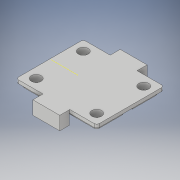
# Autodesk Inventor part: Enclosure_Top V1D5
Saved by Autodesk Inventor 2017 (Build 210142000, 142)
## iProperties
Created: 2017-12-18
Part Number: Enclosure_Top V1D5
Material: Generic
Document SubType Name: Modeling
Designer: Tripl_000
Density: 1 g/cm^3
Appearance: Default
Author: Tripl_000
Autodesk Inventor part; units mm, degrees
ref_plane "YZ Plane" through (0, 0, 0) normal (1, 0, 0) x (0, 1, 0)
ref_plane "XZ Plane" through (0, 0, 0) normal (0, 1, 0) x (-1, 0, 0)
ref_plane "XY Plane" through (0, 0, 0) normal (0, 0, 1) x (1, 0, 0)
sketch "Sketch1" plane through (0, 0, 0) normal (0, 1, 0) x (-1, 0, 0)
  line L0 (28, 23) -> (-28, 23)
  line L1 (-28, 23) -> (-28, -23)
  line L2 (-28, -23) -> (28, -23)
  line L3 (28, -23) -> (28, 23)
  line L4 (28, 23) -> (-28, -23) construction
  line L5 (-28, 23) -> (28, -23) construction
  point P0 (0, 0)
  dimension "d0" = 56
  dimension "d1" = 46
  constraints: 12 end point, 2 midpoint, 2 parallel, 1 horizontal, 1 perpendicular
  measures "d0" distance of L0.start L0.end
  measures "d1" distance of L2.end L0.start
extrude "Extrusion1" add sketch "Sketch1" along normal blind 2.5
sketch "Sketch2" plane through (0, 2.5, 0) normal (0, 1, 0) x (1, 0, 0)
  line L0 (-30, -25) -> (30, -25)
  line L1 (30, -25) -> (30, 25)
  line L2 (30, 25) -> (-30, 25)
  line L3 (-30, 25) -> (-30, -25)
  line L4 (-30, -25) -> (30, 25) construction
  line L5 (30, -25) -> (-30, 25) construction
  point P0 (0, 0)
  dimension "d4" = 50
  dimension "d5" = 60
  constraints: 12 end point, 2 midpoint, 2 parallel, 1 horizontal, 1 perpendicular
  measures "d4" distance of L2.end L0.start
  measures "d5" distance of L0.start L0.end
extrude "Extrusion2" add sketch "Sketch2" along normal blind 2.5
sketch "Sketch3" plane through (28, 0, 23) normal (1, 0, 0) x (0, 0, -1)
  line L0 (19.5, -2.5) -> (26.5, -2.5)
  line L1 (26.5, -2.5) -> (26.5, 2.5)
  line L2 (26.5, 2.5) -> (19.5, 2.5)
  line L3 (19.5, 2.5) -> (19.5, -2.5)
  line L4 (19.5, -2.5) -> (26.5, 2.5) construction
  line L5 (26.5, -2.5) -> (19.5, 2.5) construction
  point P0 (23, 0)
  dimension "d8" = 7
  dimension "d9" = 5
  constraints: 12 end point, 2 midpoint, 2 parallel, 1 horizontal, 1 perpendicular
  measures "d8" distance of L1.end L2.end
  measures "d9" distance of L0.end L1.end
extrude "Extrusion3" cut sketch "Sketch3" against normal through all
sketch "Sketch4" plane through (0, 5, 0) normal (0, 1, 0) x (1, 0, 0)
  line L0 (0, 31.16) -> (0, -35.6529)
  line L1 (-50.8705, 0) -> (45.6531, 0)
  circle A0 centre (-22.5, 17.5) radius 3.683
  circle A1 centre (22.5, 17.5) radius 3.683
  circle A2 centre (-22.5, -17.5) radius 3.683
  circle A3 centre (22.5, -17.5) radius 3.683
  point P0 (0, 0)
  dimension "d12" = 22.5
  dimension "d13" = 17.5
  dimension "d14" = 7.366
  constraints: 4 centre point, 4 end point, 3 symmetric about line, 1 horizontal, 1 vertical, 3 other
  measures "d12" horizontal distance of point (0, 0) A0.centre
  measures "d13" vertical distance of point (0, 0) A0.centre
  measures "d14" diameter of A0
fillet "Fillet1" radius 2 8 edges at (-28, 1.25, 23) (28, 1.25, 23) (28, 1.25, -23) (-28, 1.25, -23) (-30, 3.75, -25) (-30, 3.75, 25) (30, 3.75, 25) (30, 3.75, -25)
extrude "Extrusion5" cut sketch "Sketch4" against normal through all
sketch "Sketch5" plane through (-26, 0, 23) normal (0, 0, 1) x (1, 0, 0)
  line L0 (0, 2.5) -> (52, 2.5) projected
  line L1 (18.5, -2.5) -> (33.5, -2.5)
  line L2 (33.5, -2.5) -> (33.5, 2.5)
  line L3 (33.5, 2.5) -> (18.5, 2.5)
  line L4 (18.5, 2.5) -> (18.5, -2.5)
  line L5 (18.5, -2.5) -> (33.5, 2.5) construction
  line L6 (33.5, -2.5) -> (18.5, 2.5) construction
  point P0 (26, 0)
  dimension "d20" = 15
  constraints: 12 end point, 2 midpoint, 2 parallel, 1 horizontal, 1 perpendicular, 1 point on line
  measures "d20" distance of L1.start L1.end
extrude "Extrusion6" cut sketch "Sketch5" against normal through all
sketch "Sketch6" plane through (-28, 2.5, 25) normal (0, 0, 1) x (1, 0, 0)
  line L0 (20.5, 0) -> (20.5, -2.5) projected
  line L1 (56, 2.5) -> (0, 2.5) projected
  line L2 (20.5, 0) -> (35.5, 0)
  line L3 (35.5, 0) -> (35.5, 2.5)
  line L4 (35.5, 2.5) -> (20.5, 2.5)
  line L5 (20.5, 2.5) -> (20.5, 0)
  point P0 (28, -2.5)
  dimension "d23" = 15
  constraints: 8 end point, 2 parallel, 1 horizontal, 1 perpendicular, 1 point on line
  measures "d23" distance between parallel lines of L3 L5
extrude "Extrusion7" add sketch "Sketch6" along normal blind 10
sketch "Sketch7" plane through (0, 2.5, 0) normal (0, -1, 0) x (1, 0, 0)
  line L0 (-7.5, 25) -> (-7.5, 35) projected
  line L1 (7.5, 25) -> (7.5, 35) projected
  line L2 (-7.5, 35) -> (7.5, 35)
  line L3 (7.5, 35) -> (7.5, 30)
  line L4 (7.5, 30) -> (-7.5, 30)
  line L5 (-7.5, 30) -> (-7.5, 35)
  point P0 (0, 0)
  dimension "d26" = 5
  constraints: 8 end point, 2 parallel, 1 horizontal, 1 midpoint, 1 perpendicular
  measures "d26" distance between parallel lines of L4 L2
extrude "Extrusion8" add sketch "Sketch7" along normal blind 7.5
sketch "Sketch8" plane through (-7.5, 2.5, 25) normal (-1, 0, 0) x (0, 0, 1)
  line L0 (10, 2.5) -> (10, -7.5) projected
  line L1 (0, 2.5) -> (10, 2.5) projected
  line L2 (10, -7.5) -> (7.5, -7.5)
  line L3 (7.5, -7.5) -> (7.5, 2.5)
  line L4 (7.5, 2.5) -> (10, 2.5)
  line L5 (10, 2.5) -> (10, -7.5)
  point P0 (-25, -2.5)
  dimension "d29" = 2.5
  constraints: 8 end point, 2 parallel, 1 horizontal, 1 perpendicular, 1 point on line
  measures "d29" distance between parallel lines of L0 L3
extrude "Extrusion9" cut sketch "Sketch8" against normal through all
sketch "Sketch9" plane through (-7.5, -5, 32.5) normal (0, 0, 1) x (1, 0, 0)
  line L0 (0, 7.5) -> (0, 0) projected
  line L1 (35.5, 10) -> (-20.5, 10) projected
  line L2 (0, 0) -> (-2.5, 0)
  line L3 (-2.5, 0) -> (-2.5, 10)
  line L4 (-2.5, 10) -> (0, 10)
  line L5 (0, 10) -> (0, 0)
  line L6 (7.5, 20.7605) -> (7.5, -11.2566)
  line L7 (0, 0) -> (15, 0) projected
  line L8 (15, 0) -> (17.5, 0)
  line L9 (17.5, 0) -> (17.5, 10)
  line L10 (17.5, 10) -> (15, 10)
  line L11 (15, 10) -> (15, 0)
  point P0 (7.5, 5)
  dimension "d32" = 2.5
  dimension "d33" = 2.5
  constraints: 18 end point, 4 parallel, 2 horizontal, 2 perpendicular, 2 point on line, 1 vertical
  measures "d32" distance between parallel lines of L0 L3
  measures "d33" distance between parallel lines of L9 L11
extrude "Extrusion10" add sketch "Sketch9" against normal up to surface (7.5 mm away) contours L0 L2 L3 L1 L5 | L11 L1 L9 L8
ref_plane "Work Plane1" through (-28, 2.5, 0) normal (0, 0, 1) x (1, 0, 0)
mirror "Mirror1" about plane through (-28, 2.5, 0) normal (0, 0, 1) of "Extrusion7", "Extrusion8", "Extrusion9", "Extrusion10"
sketch "Sketch10" plane through (0, -5, 0) normal (0, -1, 0) x (1, 0, 0)
  line L0 (10, 25) -> (28, 25) projected
  line L1 (-10, 32.5) -> (-10, 25) projected
  line L2 (10, 25) -> (-10, 25)
  line L3 (-10, 25) -> (-10, 25.5)
  line L4 (-10, 25.5) -> (10, 25.5)
  line L5 (10, 25.5) -> (10, 25)
  line L6 (28, -25) -> (10, -25) projected
  line L7 (10, -25) -> (-10, -25)
  line L8 (-10, -25) -> (-10, -25.5)
  line L9 (-10, -25.5) -> (10, -25.5)
  line L10 (10, -25.5) -> (10, -25)
  point P0 (0, 0)
  dimension "d37" = 0.5
  dimension "d38" = 0.5
  constraints: 16 end point, 4 parallel, 2 horizontal, 2 perpendicular, 2 point on line
  measures "d37" distance between parallel lines of L4 L2
  measures "d38" distance between parallel lines of L7 L9
extrude "Extrusion11" cut sketch "Sketch10" against normal up to surface (7.5 mm away)
fillet "Fillet2" radius 5 2 edges at (0, 2.5, 30) (0, 2.5, -30)
body "Solid1"
